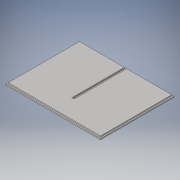
# Autodesk Inventor part: Top
Saved by Autodesk Inventor 2016 (Build 200138000, 138)
## iProperties
Created: 2017-10-30
Part Number: Top
Material: Generic
Document SubType Name: Modeling
Designer: mathaetaes
Density: 1 g/cm^3
Appearance: Default
Author: mathaetaes
Autodesk Inventor part; units mm, degrees
ref_plane "YZ Plane" through (0, 0, 0) normal (1, 0, 0) x (0, 1, 0)
ref_plane "XZ Plane" through (0, 0, 0) normal (0, 1, 0) x (-1, 0, 0)
ref_plane "XY Plane" through (0, 0, 0) normal (0, 0, 1) x (1, 0, 0)
sketch "Sketch1" plane through (0, 0, 0) normal (0, 1, 0) x (-1, 0, 0)
  line L0 (367.8783, -267.593) -> (-432.2217, -267.593)
  line L1 (-432.2217, -267.593) -> (-432.2217, 354.707)
  line L2 (-432.2217, 354.707) -> (367.8783, 354.707)
  line L3 (367.8783, 354.707) -> (367.8783, -267.593)
  point P0 (0, 0)
  dimension "d0" = 622.3
  dimension "d1" = 800.1
  constraints: 8 end point, 2 parallel, 1 horizontal, 1 perpendicular
  measures "d0" distance of L0.end L1.end
  measures "d1" distance of L1.end L2.end
extrude "Board" add sketch "Sketch1" along normal blind 19.05
sketch "Sketch3" plane through (0, 19.05, 0) normal (0, 1, 0) x (1, 0, 0)
  line L0 (432.2217, -354.707) -> (432.2217, 267.593) projected
  line L1 (22.6467, -186.432) -> (41.6967, -186.432)
  line L2 (41.6967, -186.432) -> (41.6967, 267.593)
  line L3 (41.6967, 267.593) -> (22.6467, 267.593)
  line L4 (22.6467, 267.593) -> (22.6467, -186.432)
  line L5 (432.2217, 267.593) -> (-367.8783, 267.593) projected
  line L6 (-367.8783, 267.593) -> (-367.8783, -354.707) projected
  point P0 (0, 0)
  dimension "d17" = 19.05
  dimension "d26" = 454.025
  dimension "d27" = 390.525
  constraints: 8 end point, 2 parallel, 1 collinear, 1 horizontal, 1 perpendicular
  measures "d17" distance between parallel lines of L4 L2
  measures "d26" distance of L3.end L1.start
  measures "d27" distance between parallel lines of L6 L4
extrude "Vertical Wall Dado Cuts" cut sketch "Sketch3" against normal blind 9.525
sketch "Sketch5" plane through (0, 19.05, 0) normal (0, 1, 0) x (1, 0, 0)
  line L0 (-367.8783, -354.707) -> (432.2217, -354.707) projected
  line L1 (432.2217, -354.707) -> (422.6967, -354.707)
  line L2 (422.6967, -354.707) -> (422.6967, 267.593)
  line L3 (422.6967, 267.593) -> (432.2217, 267.593)
  line L4 (432.2217, 267.593) -> (432.2217, -354.707)
  line L5 (432.2217, 267.593) -> (-367.8783, 267.593) projected
  line L6 (-367.8783, -354.707) -> (-358.3533, -354.707)
  line L7 (-358.3533, -354.707) -> (-358.3533, 267.593)
  line L8 (-358.3533, 267.593) -> (-367.8783, 267.593)
  line L9 (-367.8783, 267.593) -> (-367.8783, -354.707)
  line L10 (432.2217, 267.593) -> (-367.8783, 267.593) projected
  line L11 (432.2217, -354.707) -> (-367.8783, -354.707)
  line L12 (-367.8783, -354.707) -> (-367.8783, -345.182)
  line L13 (-367.8783, -345.182) -> (432.2217, -345.182)
  line L14 (432.2217, -345.182) -> (432.2217, -354.707)
  line L15 (-367.8783, 267.593) -> (432.2217, 267.593)
  line L16 (432.2217, 267.593) -> (432.2217, 258.068)
  line L17 (432.2217, 258.068) -> (-367.8783, 258.068)
  line L18 (-367.8783, 258.068) -> (-367.8783, 267.593)
  line L19 (432.2217, -354.707) -> (432.2217, 267.593) projected
  point P0 (0, 0)
  point P1 (422.6967, 267.593)
  point P2 (22.6467, 267.593)
  point P3 (-348.8283, 267.593)
  dimension "d22" = 9.525
  constraints: 32 end point, 8 parallel, 4 collinear, 4 horizontal, 4 perpendicular, 3 equal length
  measures "d22" distance of L2.end L3.end
extrude "Perimeter rabbit dado" cut sketch "Sketch5" against normal blind 9.525 contours L9 L13 L7 L0 | L7 L13 L2 L0 | L9 L17 L7 L13 | L2 L13 L4 L0 | L9 L5 L7 L17 | L2 L17 L4 L13 | L7 L5 L2 L17 | L2 L3 L4 L17
equation "\"d27\" = -0.5 * d17 + 0.5 * d1"
body "Solid1"
